Anschluss Abwasser Terrasse (Autodesk Fusion 360 design; units mm, degrees)
Autodesk Fusion 360 part; units mm, degrees
sketch "Sketch1" plane through (0, 0, 0) normal (0, 0, 1) x (1, 0, 0)
  circle A0 centre (0, 0) radius 74
  circle A1 centre (0, 18) radius 25.5
  circle A2 centre (0, 0) radius 70
  circle A3 centre (0, 18) radius 29
  dimension "d1" = 148
  dimension "d2" = 51
  dimension "d3" = 18
  dimension "d4" = 140
  dimension "d5" = 58
  constraint coincident A0.centre A2.centre
  constraint concentric A1 A3
  measures "d1" diameter of A0
  measures "d2" diameter of A1
  measures "d3" distance of A0.centre A1.centre
  measures "d4" diameter of A2
  measures "d5" diameter of A3
extrude "Extrude1" add sketch "Sketch1" along normal blind 5 contours A0 | A2 | A3
extrude "Extrude2" add sketch "Sketch1" along normal blind 20
fillet "Fillet1" radius 10 2 edges at (-27.0375, 28.4868, 5) (-65.2629, -25.3131, 5)
